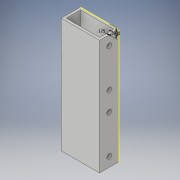
# Autodesk Inventor part: 2AM-17-P-0205
Saved by Autodesk Inventor 2017 (Build 210142000, 142)
## iProperties
Created: 2017-12-27
Part Number: 2AM-17-P-0205
Material: Generic
Document SubType Name: Modeling
Designer: Micah
Density: 1 g/cm^3
Appearance: Default
Author: Micah
Autodesk Inventor part; units mm, degrees
ref_plane "YZ Plane" through (0, 0, 0) normal (1, 0, 0) x (0, 1, 0)
ref_plane "XZ Plane" through (0, 0, 0) normal (0, 1, 0) x (-1, 0, 0)
ref_plane "XY Plane" through (0, 0, 0) normal (0, 0, 1) x (1, 0, 0)
sketch "Sketch1" plane through (0, 0, 0) normal (0, 1, 0) x (-1, 0, 0)
  line L0 (0, 0) -> (-50.8, 0)
  line L1 (-50.8, 0) -> (-50.8, -25.4)
  line L2 (-50.8, -25.4) -> (0, -25.4)
  line L3 (0, -25.4) -> (0, 0)
  line L4 (-3.175, -22.225) -> (-47.625, -22.225)
  line L5 (-47.625, -22.225) -> (-47.625, -3.175)
  line L6 (-47.625, -3.175) -> (-3.175, -3.175)
  line L7 (-3.175, -3.175) -> (-3.175, -22.225)
  dimension "d0" = 50.8
  dimension "d1" = 25.4
  dimension "d2" = 44.45
  dimension "d3" = 19.05
  dimension "d4" = 3.175
  dimension "d5" = 3.175
  constraints: 16 end point, 4 parallel, 2 horizontal, 2 perpendicular
  measures "d0" distance of L2.end L1.end
  measures "d1" distance of L1.end L0.end
  measures "d2" distance of L5.end L6.end
  measures "d3" distance of L4.end L5.end
  measures "d4" distance between parallel lines of L2 L4
  measures "d5" distance between parallel lines of L7 L3
extrude "Extrusion1" add sketch "Sketch1" along normal blind 152.4
sketch "Sketch2" plane through (0, 0, -25.4) normal (-1, 0, 0) x (0, 0, 1)
  line L0 (22.225, 152.4) -> (3.175, 152.4) projected
  line L1 (12.7, 152.4) -> (12.7, 0) construction
  line L2 (3.175, 0) -> (22.225, 0) projected
  line L3 (0, 0) -> (0, 152.4) construction
  line L4 (25.4, 0) -> (25.4, 152.4) construction
  line L5 (25.4, 0) -> (25.4, 152.4) projected
  line L6 (25.4, 76.2) -> (0, 76.2) construction
  circle A0 centre (12.7, 88.9) radius 3.175
  circle A1 centre (12.7, 63.5) radius 3.175
  circle A2 centre (12.7, 139.7) radius 3.175
  circle A3 centre (12.7, 12.7) radius 3.175
  dimension "d8" = 6.35
  dimension "d9" = 12.7
  dimension "d10" = 6.35
  dimension "d11" = 12.7
  constraints: 4 centre point, 4 end point, 4 midpoint, 2 point on line, 2 symmetric about line, 2 other
  measures "d8" diameter of A0
  measures "d9" distance from line of L6 A0.centre
  measures "d10" diameter of A2
  measures "d11" distance from line of L0 A2.centre
hole "Hole2" at (0, 139.7, -12.7) at (0, 88.9, -12.7) at (0, 63.5, -12.7) at (0, 12.7, -12.7) direction (1, 0, 0) diameter 6.35 end through all
sketch "Sketch3" plane through (50.8, 0, -25.4) normal (0, 0, -1) x (-1, 0, 0)
  line L0 (50.8, 152.4) -> (0, 152.4) projected
  line L1 (25.4, 152.4) -> (25.4, 0) construction
  line L2 (12.7, 152.4) -> (12.7, 139.7) construction
  line L3 (0, 0) -> (0, 152.4) projected
  line L4 (0, 133.35) -> (50.8, 133.35) construction
  circle A0 centre (12.7, 139.7) radius 1.5875
  circle A1 centre (38.1, 139.7) radius 1.5875
  circle A2 centre (12.7, 127) radius 1.5875
  circle A3 centre (38.1, 127) radius 1.5875
  point P0 (50.8, 0)
  dimension "d27" = 12.7
  dimension "d28" = 12.7
  dimension "d30" = 3.175
  constraints: 6 end point, 4 centre point, 3 symmetric about line, 2 point on line, 1 coincident, 1 horizontal, 1 midpoint, 1 vertical, 3 other
  measures "d27" distance of L2.start L2.end
  measures "d28" distance between parallel lines of L3 L2
  measures "d30" diameter of A0
body "Solid1"
